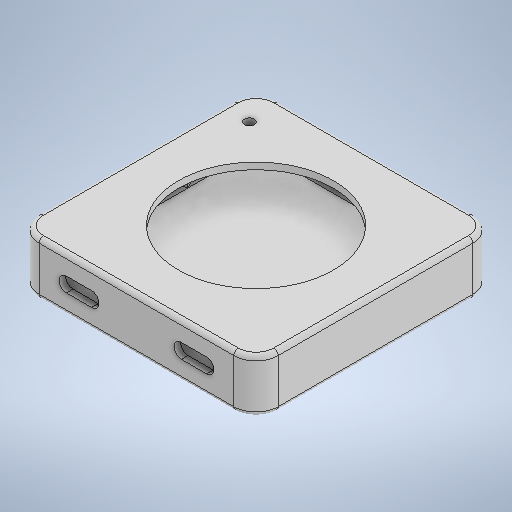
# Autodesk Inventor part: Box
Saved by Autodesk Inventor 2026 (Build 300175050, 175E)
## iProperties
Created: 2025-07-10
Part Number: Box
Material: Generic
Document SubType Name: Modeling
Designer: Jochen Alt
Density: 1 g/cm^3
Appearance: Default
Author: Jochen Alt
Autodesk Inventor part; units mm, degrees
ref_plane "YZ Plane" through (0, 0, 0) normal (1, 0, 0) x (0, 1, 0)
ref_plane "XZ Plane" through (0, 0, 0) normal (0, 1, 0) x (-1, 0, 0)
ref_plane "XY Plane" through (0, 0, 0) normal (0, 0, 1) x (1, 0, 0)
sketch "Sketch1" plane through (0, 0, 0) normal (0, 0, 1) x (1, 0, 0)
  line L0 (0, 37.8) -> (0, -37.8) construction
  line L1 (-37.8, 0) -> (37.8, 0) construction
  line L2 (-27, 27) -> (27, 27)
  line L3 (27, 27) -> (27, -27)
  line L4 (27, -27) -> (-27, -27)
  line L5 (-27, -27) -> (-27, 27)
  circle A0 centre (0, 0) radius 17.5
  dimension "d1" = 54
  dimension "d2" = 54
  dimension "d25" = 35
  constraints: 8 end point, 2 parallel, 1 centre point, 1 coincident, 1 horizontal, 1 perpendicular, 2 other
  measures "d1" distance between parallel lines of L3 L5
  measures "d2" distance between parallel lines of L4 L2
  measures "d25" diameter of A0
extrude "Extrusion1" add sketch "Sketch1" along normal blind 12 contours L2 L3 L4 L5 | A0
fillet "Fillet1" radius 5 4 edges at (-27, -27, 6) (27, -27, 6) (27, 27, 6) (-27, 27, 6)
fillet "Fillet2" radius 1 16 edges at (-25.5355, 25.5355, 12) (-27, 0, 12) (-25.5355, -25.5355, 12) (0, -27, 12) (25.5355, -25.5355, 12) (27, 0, 12) (25.5355, 25.5355, 12) (0, 27, 12) (-25.5355, 25.5355, 0) (-27, 0, 0) (-25.5355, -25.5355, 0) (0, -27, 0) (25.5355, -25.5355, 0) (27, 0, 0) (25.5355, 25.5355, 0) (0, 27, 0)
shell "Shell2" thickness 1.5 removed faces 0
sketch "USBPort" plane through (0, 0, 0) normal (0, 1, 0) x (-1, 0, 0)
  line L0 (15.85, 6) -> (10.15, 6) construction
  line L1 (15.85, 4.35) -> (10.15, 4.35)
  line L2 (10.15, 7.65) -> (15.85, 7.65)
  arc A0 (15.85, 4.35) -> (15.85, 7.65) centre (15.85, 6) ccw
  arc A1 (10.15, 7.65) -> (10.15, 4.35) centre (10.15, 6) ccw
  line L3 (-27.8, 0) -> (33.8, 0) construction
  line L4 (0, -2.1) -> (0, 12.6) construction
  circle A2 centre (-18, 6) radius 1
  line L5 (-15.85, 4.35) -> (-10.15, 4.35)
  line L6 (-10.15, 7.65) -> (-15.85, 7.65)
  arc A3 (-15.85, 7.65) -> (-15.85, 4.35) centre (-15.85, 6) ccw
  arc A4 (-10.15, 4.35) -> (-10.15, 7.65) centre (-10.15, 6) ccw
  line L7 (25.5, 1.5) -> (25.5, 10.5) projected
  point P0 (0, 0)
  point P1 (13, 6)
  point P2 (8.5, 6)
  point P3 (17.5, 6)
  point P4 (13, 7.65)
  dimension "d16" = 6
  dimension "d20" = 2
  dimension "d21" = 6
  dimension "d22" = 18
  dimension "d33" = 9
  dimension "d34" = 3.3
  dimension "d35" = 8
  constraints: 12 end point, 10 point on circle, 6 symmetric about line, 5 centre point, 4 tangent, 2 midpoint, 1 horizontal, 1 parallel, 2 other
  measures "d16" distance between parallel lines of L3 L0
  measures "d20" diameter of A2
  measures "d21" distance from line of L3 A2.centre
  measures "d22" distance from line of L4 A2.centre
  measures "d33" distance of point (8.5, 6) point (17.5, 6)
  measures "d34" distance from line of L1 point (13, 7.65)
  measures "d35" distance from line of point (17.5, 6) L7
extrude "USB Port" cut sketch "USBPort" against normal up to next contours L1 A1 L2 A0 | A2 A3 | A2 A3 L6 A4 L5 picked at (-17.3258, 6.1952)
extrude "Extrusion5" cut sketch "USBPort" along normal up to next contours A2 A3 | A3 A2
extrude "Extrusion6" cut sketch "Sketch1" against normal blind 5 from surface at 12 contours A0
sketch "LED" plane through (0, 0, 0) normal (0, 0, 1) x (1, 0, 0)
  line L0 (0, 37.1) -> (0, -37.1) construction
  line L1 (-37.1, 0) -> (37.1, 0) construction
  line L2 (-27, 27) -> (27, 27) construction
  line L3 (-27, -27) -> (-27, 27) construction
  line L4 (27, -27) -> (-27, -27) construction
  line L5 (27, 27) -> (27, -27) construction
  line L6 (-22, -25.5) -> (22, -25.5) projected
  line L7 (-22.5, 7) -> (-19.5, 7)
  line L8 (-19.5, 7) -> (-19.5, 4)
  line L9 (-19.5, 4) -> (-22.5, 4)
  line L10 (-22.5, 4) -> (-22.5, 7)
  line L11 (-22.5, 7) -> (-19.5, 4) construction
  line L12 (-22.5, 4) -> (-19.5, 7) construction
  circle A0 centre (-21, 19.5) radius 1.1
  line L13 (-22.5, 21) -> (-19.5, 21) construction
  line L14 (-19.5, 21) -> (-19.5, 18)
  line L15 (-19.5, 18) -> (-22.5, 18)
  line L16 (-22.5, 18) -> (-22.5, 21)
  line L17 (-22.5, 21) -> (-19.5, 18) construction
  line L18 (-19.5, 21) -> (-22.5, 18) construction
  line L19 (-21, 19.5) -> (-21, 5.5) construction
  line L20 (-22.5, 21) -> (-22.5, 22.5)
  line L21 (-22.5, 22.5) -> (-19.5, 22.5)
  line L22 (-19.5, 22.5) -> (-19.5, 21)
  line L23 (19, 25.5) -> (17, 25.5) construction
  line L24 (-22, 25.5) -> (22, 25.5) construction
  line L25 (-22, 25.5) -> (22, 25.5) construction
  line L26 (-25.5, -22) -> (-25.5, 22) construction
  line L27 (-25.5, 22) -> (-25.5, -22) construction
  point P0 (0, 0)
  point P1 (-21, 19.5)
  dimension "d37" = 3
  dimension "d38" = 2.2
  dimension "d40" = 3
  dimension "d41" = 6
  dimension "d42" = 31
  dimension "d53" = 1.5
  dimension "d56" = 6
  constraints: 32 end point, 7 perpendicular, 5 midpoint, 5 parallel, 2 horizontal, 1 centre point, 1 coincident, 1 vertical
  measures "d37" distance of L8.end L9.end
  measures "d38" diameter of A0
  measures "d40" distance of L14.end L15.end
  measures "d41" distance between parallel lines of L19 L3
  measures "d42" distance from line of L6 point (-21, 5.5)
  measures "d53" distance of L13.start L20.end
  measures "d56" distance from line of L24 point (-21, 19.5)
extrude "Extrusion8" add sketch "LED" against normal blind 3 from surface at 10.5 contours L7 L8 L9 L10
chamfer "Chamfer1" distance 3 angle 45 1 edges at (-21, 7, 7.5)
extrude "Extrusion9" add sketch "LED" against normal blind 3 from surface at 10.5 separate body contours A0 | L14 L15 L16 L20 L21 L22
chamfer "Chamfer2" distance 3 angle 45 1 edges at (-21, 18, 10.5)
combine bodies "Combine1" operation type add bodies to combine 2 1
extrude "Extrusion10" cut sketch "LED" against normal blind 2 from surface at 12 contours A0 bodies 2
equation "\"d2\" = d1"
equation "\"d21\" = d16"
equation "\"d56\" = d41"
body "Solid2"
